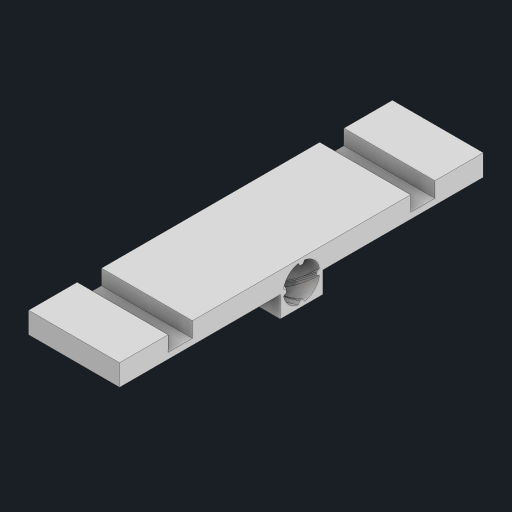
# Autodesk Inventor part: screw_slider
Saved by Autodesk Inventor 2024 (Build 280153000, 153)
## iProperties
Created: 2024-06-23
Part Number: screw_slider
Material: Generic
Document SubType Name: Modeling
Designer: mihir
Density: 1 g/cm^3
Appearance: Default
Author: mihir
Autodesk Inventor part; units mm, degrees
ref_plane "YZ Plane" through (0, 0, 0) normal (1, 0, 0) x (0, 1, 0)
ref_plane "XZ Plane" through (0, 0, 0) normal (0, 1, 0) x (-1, 0, 0)
ref_plane "XY Plane" through (0, 0, 0) normal (0, 0, 1) x (1, 0, 0)
sketch "Sketch1" plane through (0, 0, 0) normal (0, 1, 0) x (-1, 0, 0)
  line L0 (0, 0) -> (30, 0)
  line L1 (30, 0) -> (30, -120)
  line L2 (30, -120) -> (0, -120)
  line L3 (0, -120) -> (0, 0)
  dimension "d0" = 120
  dimension "d1" = 30
  constraints: 8 end point, 2 parallel, 1 horizontal, 1 perpendicular
  measures "d0" distance of L2.end L0.start
  measures "d1" distance of L0.start L0.end
extrude "Extrusion1" add sketch "Sketch1" along normal blind 7
sketch "Sketch2" plane through (0, 0, 0) normal (0, -1, 0) x (1, 0, 0)
  line L0 (-5, -5) -> (-25, -5)
  line L1 (-25, -5) -> (-25, -10)
  line L2 (-25, -10) -> (-5, -10)
  line L3 (-5, -10) -> (-5, -5)
  line L4 (-30, 0) -> (0, 0) projected
  line L5 (0, 0) -> (0, -120) projected
  line L6 (0, 0) -> (0, -120) construction
  line L7 (0, -40) -> (-30, -40) construction
  line L8 (-30, -120) -> (-30, 0) construction
  dimension "d4" = 5
  dimension "d5" = 20
  dimension "d6" = 5
  dimension "d7" = 5
  dimension "d8" = 40
  constraints: 10 end point, 2 horizontal, 2 parallel, 2 point on line, 1 perpendicular
  measures "d4" distance of L2.end L0.start
  measures "d5" distance of L0.start L0.end
  measures "d6" distance between parallel lines of L4 L0
  measures "d7" distance between parallel lines of L5 L3
  measures "d8" distance between parallel lines of L4 L7
revolve "Revolution1" cut sketch "Sketch2" angle 360 about axis through (-25, 0, -10) along (1, 0, 0)
sketch "Sketch3" plane through (0, 0, 0) normal (0, -1, 0) x (1, 0, 0)
  line L0 (0, 0) -> (0, -120) construction
  line L1 (0, -40) -> (-30, -40) construction
  line L2 (-30, -120) -> (-30, 0) construction
  line L3 (-30, 0) -> (0, 0) construction
  line L4 (-10, -20) -> (-20, -20) construction
  line L5 (-15, -20) -> (-15, -40) construction
  dimension "d10" = 40
  dimension "d11" = 20
  dimension "d12" = 10
  constraints: 6 end point, 2 horizontal, 2 midpoint, 2 point on line, 1 vertical
  measures "d10" distance between parallel lines of L3 L1
  measures "d11" distance of L5.start L5.end
  measures "d12" distance of L4.end L4.start
hole "Hole1" at (-10, 0, -20) at (-20, 0, -20) direction (0, 1, 0) diameter 1 depth 7 tip angle 118
sketch "Sketch4" plane through (0, 7, 0) normal (0, 1, 0) x (1, 0, 0)
  line L0 (-5, 15) -> (-25, 15) projected
  line L1 (-25, 15) -> (-25, 5) projected
  line L2 (-30, 120) -> (-30, 0) projected
  line L3 (0, 0) -> (0, 120) projected
  line L4 (-30, 16) -> (0, 16)
  line L5 (0, 16) -> (0, 24)
  line L6 (0, 24) -> (-30, 24)
  line L7 (-30, 24) -> (-30, 16)
  line L8 (-30, 20) -> (0, 20) construction
  circle A0 centre (-20, 20) radius 0.5 construction
  circle A1 centre (-10, 20) radius 0.5 construction
  line L9 (-20, 20) -> (-10, 20) construction
  point P0 (-30, 24)
  point P1 (0, 16)
  dimension "d20" = 8
  constraints: 12 end point, 2 horizontal, 2 midpoint, 2 parallel, 2 point on line, 1 collinear, 1 perpendicular
  measures "d20" distance between parallel lines of L4 L6
extrude "Extrusion2" cut sketch "Sketch4" against normal blind 5
ref_plane "Work Plane1" through (-30, 0, -60) normal (0, 0, 1) x (1, 0, 0)
mirror "Mirror1" about plane through (-30, 0, -60) normal (0, 0, 1) of "Revolution1", "Hole1", "Extrusion2"
sketch "Sketch5" plane through (0, 0, 0) normal (1, 0, 0) x (0, 0, -1)
  circle A0 centre (60, 0) radius 6
  line L0 (0, 0) -> (120, 0) projected
  line L1 (24, 7) -> (96, 7) projected
  line L2 (53, -7) -> (67, -7)
  line L3 (67, -7) -> (67, 7)
  line L4 (67, 7) -> (53, 7)
  line L5 (53, 7) -> (53, -7)
  line L6 (53, -7) -> (67, 7) construction
  line L7 (67, -7) -> (53, 7) construction
  point P0 (67, 0)
  point P1 (66, 0)
  point P2 (54, 0)
  point P3 (53, 0)
  dimension "d23" = 12
  constraints: 12 end point, 3 midpoint, 2 parallel, 2 perpendicular, 1 centre point, 1 coincident, 1 horizontal, 1 point on line
  measures "d23" diameter of A0
extrude "Extrusion3" add sketch "Sketch5" against normal up to surface (30 mm away) contours L0 L3 L2 L5 A0
sketch "Sketch6" plane through (0, 0, -120) normal (1, 0, 0) x (0, 0, -1)
  line L0 (-54, 0) -> (-66, 0) projected
  arc A0 (-54, 0) -> (-66, 0) centre (-60, 0) ccw
  line L1 (-66, 0) -> (-54, 0)
  point P0 (-120, 0)
  constraints: 2 end point, 2 point on circle, 1 centre point, 1 collinear, 1 midpoint
extrude "Extrusion4" cut sketch "Sketch6" against normal up to surface (30 mm away)
sketch "Sketch7" plane through (0, 0, -120) normal (1, 0, 0) x (0, 0, -1)
  circle A0 centre (-60, 0) radius 6 construction
  circle A1 centre (-60, 0) radius 5 construction
  line L0 (-65, 0) -> (-65, 0.5)
  line L1 (-65, 0.5) -> (-66, 1.0774)
  line L2 (-66, 1.0774) -> (-66, 0)
  line L3 (-66, 0) -> (-65, 0)
  line L4 (-65, 0) -> (-65, -0.5)
  line L5 (-65, -0.5) -> (-66, -1.0774)
  line L6 (-66, -1.0774) -> (-66, 0)
  point P0 (-120, 0)
  dimension "d28" = 10
  dimension "d29" = 120
  dimension "d30" = 0.5
  constraints: 14 end point, 3 vertical, 2 horizontal alignment, 2 symmetric about line, 1 coincident, 1 horizontal, 3 other
  measures "d30" distance of L0.start L0.end
coil "Coil1" sketch "Sketch7" operation add axis through (0, 0, -60) along (-1, 0, 0) pitch 40 turns 0.75 hand right
pattern_circular "Circular Pattern1" count 4 over 360 about axis through (0, 0, -60) along (-1, 0, 0) of "Coil1"
equation "\"d0\" = table_bed_width"
equation "\"d1\" = table_bed_peg_width"
equation "\"d2\" = screw_slider_thickness"
equation "\"d4\" = 0.5 * bearing_diameter"
equation "\"d5\" = bearing_length"
equation "\"d6\" = 0.5 * table_bed_peg_width - 0.5 * bearing_length"
equation "\"d7\" = 0.5 * table_bed_peg_width - 0.5 * bearing_length"
equation "\"d8\" = table_bed_peg_length"
equation "\"d10\" = table_bed_peg_length"
equation "\"d11\" = screw_y"
equation "\"d12\" = screw_x"
equation "\"d13\" = screw_diameter"
equation "\"d20\" = cutout_width"
equation "\"d23\" = lead_screw_outer_diameter"
equation "\"d28\" = lead_screw_diameter"
equation "\"d29\" = screw_profile_angle"
equation "\"d30\" = 0.5 * screw_profile_width"
equation "\"d31\" = screw_pitch"
equation "\"table_bed_width\" = 120"
equation "\"table_bed_peg_width\" = 30"
equation "\"screw_slider_thickness\" = 7"
equation "\"bearing_length\" = 20"
equation "\"table_bed_peg_length\" = 40"
equation "\"screw_y\" = 20"
equation "\"screw_x\" = 10"
equation "\"screw_diameter\" = 1"
equation "\"cutout_width\" = 8"
equation "\"lead_screw_outer_diameter\" = 12"
equation "\"screw_profile_width\" = 1"
equation "\"screw_profile_angle\" = 120deg"
equation "\"screw_pitch\" = 40"
equation "\"bearing_diameter\" = 10"
equation "\"lead_screw_diameter\" = 10"
body "Solid1"
